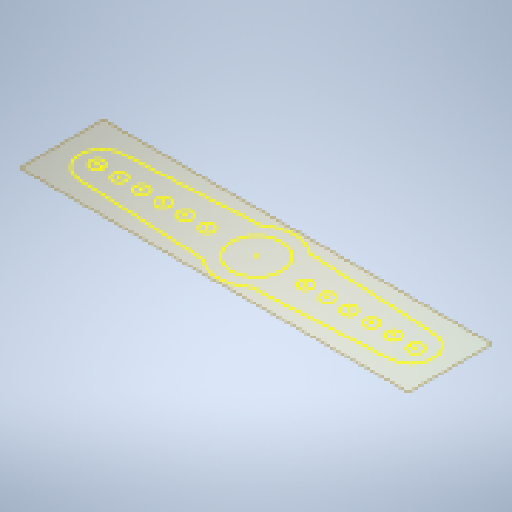
# Autodesk Inventor part: klesce1
Saved by Autodesk Inventor 2024 (Build 280153000, 153)
## iProperties
Created: 2023-09-09
Part Number: klesce1
Material: Generic
Document SubType Name: Modeling
Designer: jebes windows
Density: 1 g/cm^3
Appearance: Default
Author: jebes windows
Autodesk Inventor part; units mm, degrees
ref_plane "YZ Plane" through (0, 0, 0) normal (1, 0, 0) x (0, 1, 0)
ref_plane "XZ Plane" through (0, 0, 0) normal (0, 1, 0) x (-1, 0, 0)
ref_plane "XY Plane" through (0, 0, 0) normal (0, 0, 1) x (1, 0, 0)
ref_plane "Work Plane1" through (0, 0, 0) normal (0, 0, 1) x (1, 0, 0)
sketch "Sketch1" plane through (0, 0, 0) normal (0, 0, 1) x (1, 0, 0)
  line L0 (14.1591, 1.997) -> (2.2091, 2.65) projected
  arc A0 (2.2091, 2.65) -> (-2.2091, 2.65) centre (0, 0) ccw projected
  line L1 (-2.2091, 2.65) -> (-14.1591, 1.997) projected
  arc A1 (-14.1591, 1.997) -> (-14.1591, -1.997) centre (-14.05, 0) ccw projected
  line L2 (-14.1591, -1.997) -> (-2.2091, -2.65) projected
  arc A2 (-2.2091, -2.65) -> (2.2091, -2.65) centre (0, 0) ccw projected
  line L3 (2.2091, -2.65) -> (14.1591, -1.997) projected
  arc A3 (14.1591, -1.997) -> (14.1591, 1.997) centre (14.05, 0) ccw projected
  circle A4 centre (12.45, 0) radius 0.6 projected
  circle A5 centre (14.45, 0) radius 0.6 projected
  circle A6 centre (10.45, 0) radius 0.6 projected
  circle A7 centre (8.45, 0) radius 0.6 projected
  circle A8 centre (6.45, 0) radius 0.6 projected
  circle A9 centre (4.45, 0) radius 0.6 projected
  circle A10 centre (0, 0) radius 2.3 projected
  circle A11 centre (-4.45, 0) radius 0.6 projected
  circle A12 centre (-6.45, 0) radius 0.6 projected
  circle A13 centre (-8.45, 0) radius 0.6 projected
  circle A14 centre (-10.45, 0) radius 0.6 projected
  circle A15 centre (-12.45, 0) radius 0.6 projected
  circle A16 centre (-14.45, 0) radius 0.6 projected
  line L4 (12.5, 16.5) -> (-12.5, 16.5)
  line L5 (-12.5, 16.5) -> (-12.5, -16.5)
  line L6 (-12.5, -16.5) -> (12.5, -16.5)
  line L7 (12.5, -16.5) -> (12.5, 16.5)
  line L8 (12.5, 16.5) -> (-12.5, -16.5) construction
  line L9 (-12.5, 16.5) -> (12.5, -16.5) construction
  point P0 (0, 0)
  dimension "d0" = 33
  dimension "d1" = 25
  constraints: 12 end point, 2 midpoint, 2 parallel, 1 horizontal, 1 perpendicular
  measures "d0" distance of L5.end L4.end
  measures "d1" distance between parallel lines of L5 L7
extrude "Extrusion1" add sketch "Sketch1" along normal blind 6 contours L7 A4 L3 A2 L2 L5 A15 L1 A0 L0 | L0 A0 L1 L5 L4 L7 | L7 A4 | L7 L6 L5 L2 A2 L3 | A15 L5 | A6 | A7 | A13 | A14 picked at (12.3149, 0.1993) picked at (-12.1464, 0.1302)
sketch "Sketch2" plane through (0, 0, 6) normal (0, 0, 1) x (1, 0, 0)
  circle A0 centre (6.45, 0) radius 0.6 projected
  circle A1 centre (6.45, 0) radius 2.5
  circle A2 centre (-6.45, 0) radius 0.6 projected
  circle A3 centre (-6.45, 0) radius 2.5
  line L0 (6.45, 2.5) -> (-6.45, 2.5)
  line L1 (6.45, -2.5) -> (-6.45, -2.5)
  point P0 (0, 0)
  dimension "d4" = 5
  dimension "d5" = 5
  dimension "d6" = 12.9
  dimension "d7" = 12.9
  constraints: 4 end point, 4 point on circle, 2 centre point, 2 coincident, 2 tangent
  measures "d4" diameter of A1
  measures "d5" diameter of A3
  measures "d6" distance of L1.start L1.end
  measures "d7" distance of L0.start L0.end
extrude "Extrusion2" cut sketch "Sketch2" against normal blind 3 contours A0 | A1 | A1 L1 A3 L0 | A3 | A2
body "Solid1"
